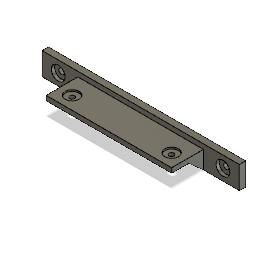
iMac HDD Holder (Autodesk Fusion 360 design; units mm, degrees)
Autodesk Fusion 360 part; units mm, degrees
sketch "Sketch1" plane through (0, 0, 0) normal (0, 0, 1) x (1, 0, 0)
  circle A0 centre (-40.7833, 0) radius 4.25
  circle A1 centre (60.2167, 0) radius 1.65
  circle A2 centre (60.2167, 0) radius 4.25
  circle A3 centre (19.2167, 0) radius 1.65
  circle A4 centre (19.2167, 0) radius 4.25
  circle A5 centre (-40.7833, 0) radius 1.65
  line L0 (-50.7833, -7) -> (70.2167, -7)
  line L1 (70.2167, -7) -> (70.2167, 7)
  line L2 (70.2167, 7) -> (-50.7833, 7)
  line L3 (-50.7833, 7) -> (-50.7833, -7)
  dimension "d3" = 8.5
  dimension "d4" = 3.3
  dimension "d5" = 8.5
  dimension "d6" = 3.3
  dimension "d7" = 8.5
  dimension "d8" = 60
  dimension "d9" = 41
  dimension "d10" = 3.3
  dimension "d11" = 14
  dimension "d12" = 10
  dimension "d13" = 10
  dimension "d14" = 7
  constraint concentric A1 A2
  constraint concentric A3 A4
  constraint horizontal origin A0.centre
  constraint horizontal origin A3.centre
  constraint horizontal origin A1.centre
  constraint concentric A0 A5
  constraint horizontal L0
  constraint vertical L1
  constraint horizontal L2
  constraint vertical L3
  measures "d3" diameter of A0
  measures "d4" diameter of A1
  measures "d5" diameter of A2
  measures "d6" diameter of A3
  measures "d7" diameter of A4
  measures "d8" distance of A0.centre A3.centre
  measures "d9" horizontal distance of A1.centre A3.centre
  measures "d10" diameter of A5
  measures "d11" distance of L0.start L2.end
  measures "d12" distance of A0.centre L3
  measures "d13" distance of A1.centre L1
  measures "d14" distance of A0.centre L2
extrude "Extrude1" add sketch "Sketch1" along normal blind 2 contours A0 | A2 makes body 1 at (-36.5386, -0.2118, 1.3333) makes body 2 at (64.4614, -0.2118, 1.3333)
extrude "Extrude2" add sketch "Sketch1" along normal blind 4 contours A3 | A4 | L0 L1 L2 L3 bodies 1 2
sketch "Sketch2" plane through (0, 0, 0) normal (0, 1, 0) x (1, 0, 0)
  circle A0 centre (-20.7833, -15.5) radius 1.5
  circle A1 centre (-20.7833, -15.5) radius 4.25
  line L0 (70.2167, 0) -> (-50.7833, 0)
  circle A2 centre (40.2167, -15.5) radius 1.5
  circle A3 centre (40.2167, -15.5) radius 4.25
  line L1 (-28.7833, -23.5) -> (48.2167, -23.5)
  line L2 (48.2167, -23.5) -> (48.2167, -4)
  line L3 (48.2167, -4) -> (-28.7833, -4)
  line L4 (-28.7833, -4) -> (-28.7833, -23.5)
  line L5 (70.2167, -4) -> (-50.7833, -4)
  point P0 (-50.7833, 0)
  point P1 (70.2167, 0)
  dimension "d19" = 3
  dimension "d20" = 8.5
  dimension "d21" = 15.5
  dimension "d22" = 3
  dimension "d23" = 8.5
  dimension "d24" = 15.5
  dimension "d25" = 30
  dimension "d27" = 8
  dimension "d28" = 8
  dimension "d29" = 8
  dimension "d36" = 61
  constraint concentric A0 A1
  constraint concentric A2 A3
  constraint horizontal L1
  constraint vertical L2
  constraint horizontal L3
  constraint vertical L4
  constraint collinear L3 L5
  measures "d19" diameter of A0
  measures "d20" diameter of A1
  measures "d21" distance of A0.centre L0
  measures "d22" diameter of A2
  measures "d23" diameter of A3
  measures "d24" distance of L0 A2.centre
  measures "d25" horizontal distance of A0.centre P0
  measures "d27" distance of A0.centre L1
  measures "d28" distance of A2.centre L2
  measures "d29" distance of A0.centre L4
  measures "d36" distance of A0.centre A2.centre
extrude "Extrude3" add sketch "Sketch2" along normal blind 3 from surface at 1 contours L1 L2 L3 L4 L5 bodies 1
extrude "Extrude4" add sketch "Sketch2" along normal blind 2 from surface at 1 contours A1 | A3 bodies 1
chamfer "Chamfer1" distance 8 distance2 9 1 edges at (9.7167, 1, 4) measured on face at (68.3001, 0, 4) on bodies 1
